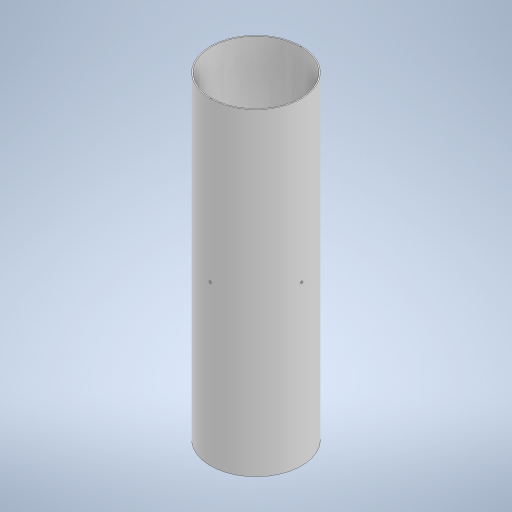
# Autodesk Inventor part: seed_holder
Saved by Autodesk Inventor 2023 (Build 270158000, 158)
## iProperties
Created: 2022-06-17
Part Number: seed_holder
Material: Generic
Document SubType Name: Modeling
Designer: prana_p9lsmih
Density: 1 g/cm^3
Appearance: Default
Author: prana_p9lsmih
Autodesk Inventor part; units mm, degrees
sketch "Sketch3" plane through (0, 0, 0) normal (0, 1, 0) x (-1, 0, 0)
  circle A0 centre (0, 0) radius 43
  circle A1 centre (0, 0) radius 42
  dimension "d8" = 86
  dimension "d9" = 84
  constraints: 2 centre point, 2 coincident
  measures "d8" diameter of A0
  measures "d9" diameter of A1
extrude "Extrusion3" add sketch "Sketch3" along normal blind 300
ref_plane "Work Plane2" through (0, 150, 0) normal (0, 1, 0) x (-1, 0, 0)
sketch "Sketch4" plane through (0, 300, 0) normal (0, 1, 0) x (1, 0, 0)
  circle A0 centre (0, 42.5) radius 0.25
  point P0 (0, 0)
  dimension "d12" = 0.5
  dimension "d13" = 42.5
  constraints: 1 centre point
  measures "d12" diameter of A0
  measures "d13" distance of point (0, 0) A0.centre
extrude "Extrusion4" cut sketch "Sketch4" along normal through all both and the other way through all
mirror "Mirror1" about plane through (0, 0, 0) normal (0, 0, 1) of "Extrusion4"
ref_plane "Work Plane3" through (43, 0, 0) normal (1, 0, 0) x (0, 1, 0)
sketch "Sketch5" plane through (43, 0, 0) normal (1, 0, 0) x (0, 1, 0)
  circle A0 centre (150, 0) radius 1
  point P0 (0, 0)
  dimension "d16" = 2
  constraints: 1 centre point
  measures "d16" diameter of A0
extrude "Extrusion5" cut sketch "Sketch5" against normal through all
ref_plane "Work Plane4" through (0, 0, 43) normal (0, 0, 1) x (1, 0, 0)
sketch "Sketch6" plane through (0, 0, 43) normal (0, 0, 1) x (1, 0, 0)
  circle A0 centre (-0.25, 150) radius 1
  point P0 (0, 0)
  constraints: 1 centre point
extrude "Extrusion6" cut sketch "Sketch6" against normal through all
body "Solid2"
